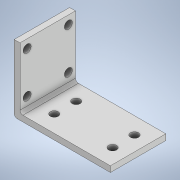
# Autodesk Inventor part: L_connector_actuators_endeffector
Saved by Autodesk Inventor 2021 (Build 250183000, 183)
## iProperties
Created: 2020-05-19
Part Number: L_connector_actuators_endeffector
Material: Generic
Document SubType Name: Modeling
Designer: Motius
Density: 1 g/cm^3
Appearance: Default
Author: Motius
Autodesk Inventor part; units mm, degrees
ref_plane "YZ Plane" through (0, 0, 0) normal (1, 0, 0) x (0, 1, 0)
ref_plane "XZ Plane" through (0, 0, 0) normal (0, 1, 0) x (-1, 0, 0)
ref_plane "XY Plane" through (0, 0, 0) normal (0, 0, 1) x (1, 0, 0)
sketch "Sketch1" plane through (0, 0, 0) normal (0, 0, 1) x (1, 0, 0)
  line L0 (-19.6971, 0) -> (73.2828, 0) construction
  line L1 (0, 49.2828) -> (0, -15.6971) construction
  line L2 (-6, 40) -> (-6, -4)
  line L3 (-4, -6) -> (60, -6)
  line L4 (60, -6) -> (60, -2)
  line L5 (60, -2) -> (0, -2)
  line L6 (-2, 0) -> (-2, 40)
  line L7 (-2, 40) -> (-6, 40)
  arc A0 (-2, 0) -> (0, -2) centre (0, 0) ccw
  arc A1 (-6, -4) -> (-4, -6) centre (-4, -4) ccw
  dimension "d0" = 2
  dimension "d1" = 4
  dimension "d2" = 4
  dimension "d3" = 40
  dimension "d5" = 60
  constraints: 12 end point, 4 point on circle, 4 tangent, 3 perpendicular, 2 centre point, 2 point on line, 1 equal radius, 1 horizontal, 1 parallel, 1 vertical
  measures "d0" radius of A0
  measures "d1" distance of L6.end L2.start
  measures "d2" distance of L3.end L4.end
  measures "d3" distance from line of L6.start L7
  measures "d5" distance from line of L4 L5.end
extrude "Extrusion1" add sketch "Sketch1" along normal mid plane 38
sketch "Sketch2" plane through (-2, 0, 19) normal (1, 0, 0) x (0, 0, -1)
  line L0 (0, 40) -> (38, 40) construction
  line L1 (0, 0) -> (0, 40) construction
  line L2 (38, 0) -> (0, 0) construction
  line L3 (38, 40) -> (38, 0) construction
  line L4 (0, 0) -> (0, 40) construction
  line L5 (0, 20) -> (38, 20) construction
  line L6 (19, 0) -> (19, 40) construction
  line L7 (0, 40) -> (38, 40) construction
  circle A0 centre (19, 20) radius 20 construction
  point P0 (33.1421, 5.8579)
  point P1 (33.1421, 34.1421)
  point P2 (4.8579, 5.8579)
  point P3 (4.8579, 34.1421)
  dimension "d17" = 40
  dimension "d18" = 28.2843
  dimension "d19" = 28.2843
  constraints: 4 end point, 4 midpoint, 4 point on circle, 4 symmetric about line, 1 centre point
  measures "d17" diameter of A0
  measures "d18" distance of A0.start point (4.858, 5.858)
  measures "d19" distance of point (4.858, 34.142) point (4.858, 5.858)
hole "Hole1" at (-2, 5.8579, -14.1421) at (-2, 34.1421, -14.1421) at (-2, 5.8579, 14.1421) at (-2, 34.1421, 14.1421) direction (-1, 0, 0) diameter 5.5 end through all clearance for "Socket Head Cap Screw" size "M5" standard "Ansi Metric M Profile"
sketch "Sketch3" plane through (-4, -6, 19) normal (0, -1, 0) x (1, 0, 0)
  line L0 (64, -38) -> (64, 0) construction
  line L1 (0, 0) -> (64, 0) construction
  line L2 (0, -38) -> (0, 0) construction
  line L3 (64, -38) -> (0, -38) construction
  line L4 (64, -19) -> (0, -19) construction
  line L5 (0, -38) -> (0, 0) construction
  line L6 (64, 0) -> (4, 0) construction
  line L7 (4, -38) -> (64, -38) construction
  line L8 (54, -11.5) -> (14, -11.5) construction
  line L9 (14, -11.5) -> (14, -26.5) construction
  line L10 (14, -26.5) -> (54, -26.5) construction
  line L11 (54, -26.5) -> (54, -11.5) construction
  line L12 (64, -38) -> (0, -38) construction
  line L13 (2, 0) -> (-2, 0) construction
  line L14 (4, -38) -> (4, 0) construction
  line L15 (34, 0) -> (34, -38) construction
  point P0 (4, -19)
  dimension "d20" = 15
  dimension "d21" = 40
  constraints: 14 end point, 4 coincident, 3 midpoint, 3 parallel, 1 horizontal, 1 perpendicular, 1 point on line, 1 vertical, 2 other
  measures "d20" distance of L10.end L8.start
  measures "d21" distance of L9.end L10.end
hole "Hole2" at (50, -6, 7.5) at (50, -6, -7.5) at (10, -6, -7.5) at (10, -6, 7.5) direction (0, 1, 0) diameter 5.5 end through all clearance for "Socket Head Cap Screw" size "M5" standard "Ansi Metric M Profile"
equation "\"d18\" = d19"
body "Solid1"
